Autodesk Inventor part; units mm, degrees
(part 2 of 2)
  arc A534 (23.3689, 24.3508) -> (23.2778, 24.4378) centre (0, 0) ccw
  arc A535 (23.1753, 25.0231) -> (23.2778, 24.4378) centre (23.6226, 24.7999) ccw
  arc A536 (23.5592, 25.726) -> (23.1753, 25.0231) centre (32.8115, 20.2148) ccw
  arc A537 (23.5592, 25.726) -> (23.6135, 25.8342) centre (22.847, 26.1505) ccw
  arc A538 (23.6135, 25.8342) -> (23.96, 26.7897) centre (12.8293, 30.2854) ccw
  arc A539 (23.96, 26.7897) -> (23.931, 26.8943) centre (23.8646, 26.8196) ccw
  arc A540 (23.931, 26.8943) -> (23.4386, 27.3246) centre (0, 0) ccw
  arc A541 (23.4386, 27.3246) -> (23.331, 27.3392) centre (23.3735, 27.2487) ccw
  arc A542 (23.331, 27.3392) -> (22.4306, 26.8676) centre (28.2892, 16.7785) ccw
  arc A543 (22.4306, 26.8676) -> (22.3307, 26.7993) centre (22.847, 26.1505) ccw
  arc A544 (21.6857, 26.3244) -> (22.3307, 26.7993) centre (15.6275, 35.228) ccw
  arc A545 (21.092, 26.3475) -> (21.6857, 26.3244) centre (21.4045, 26.7378) ccw
  arc A546 (21.092, 26.3475) -> (20.9935, 26.426) centre (0, 0) ccw
  arc A547 (20.8389, 26.9998) -> (20.9935, 26.426) centre (21.3045, 26.8175) ccw
  arc A548 (21.1584, 27.7342) -> (20.8389, 26.9998) centre (30.8673, 23.0746) ccw
  arc A549 (21.1584, 27.7342) -> (21.2027, 27.8469) centre (20.4109, 28.0932) ccw
  arc A550 (21.2027, 27.8469) -> (21.4621, 28.8296) centre (10.0629, 31.3135) ccw
  arc A551 (21.4621, 28.8296) -> (21.4239, 28.9312) centre (21.3644, 28.8509) ccw
  arc A552 (21.4239, 28.9312) -> (20.8949, 29.3156) centre (0, 0) ccw
  arc A553 (20.8949, 29.3156) -> (20.7864, 29.3205) centre (20.8368, 29.2342) ccw
  arc A554 (20.7864, 29.3205) -> (19.932, 28.7701) centre (26.6713, 19.2468) ccw
  arc A555 (19.932, 28.7701) -> (19.8385, 28.6931) centre (20.4109, 28.0932) ccw
  arc A556 (19.2387, 28.1624) -> (19.8385, 28.6931) centre (12.4067, 36.487) ccw
  arc A557 (18.6453, 28.1321) -> (19.2387, 28.1624) centre (18.9215, 28.5489) ccw
  arc A558 (18.6453, 28.1321) -> (18.5402, 28.2015) centre (0, 0) ccw
  arc A559 (18.3348, 28.7591) -> (18.5402, 28.2015) centre (18.8148, 28.6193) ccw
  arc A560 (18.5871, 29.5192) -> (18.3348, 28.7591) centre (28.6747, 25.7486) ccw
  arc A561 (18.5871, 29.5192) -> (18.6211, 29.6353) centre (17.8105, 29.8098) ccw
  arc A562 (18.6211, 29.6353) -> (18.7914, 30.6374) centre (7.2155, 32.0894) ccw
  arc A563 (18.7914, 30.6374) -> (18.7443, 30.7352) centre (18.6922, 30.6498) ccw
  arc A564 (18.7443, 30.7352) -> (18.1829, 31.0706) centre (0, 0) ccw
  arc A565 (18.1829, 31.0706) -> (18.0745, 31.0657) centre (18.1324, 30.9843) ccw
  arc A566 (18.0745, 31.0657) -> (17.2728, 30.4409) centre (24.8386, 21.5601) ccw
  arc A567 (17.2728, 30.4409) -> (17.1866, 30.3559) centre (17.8105, 29.8098) ccw
  arc A568 (16.6368, 29.7735) -> (17.1866, 30.3559) centre (9.0861, 37.4523) ccw
  arc A569 (16.0485, 29.6902) -> (16.6368, 29.7735) centre (16.2863, 30.1301) ccw
  arc A570 (16.0485, 29.6902) -> (15.9376, 29.7499) centre (0, 0) ccw
  arc A571 (15.683, 30.2868) -> (15.9376, 29.7499) centre (16.1737, 30.1906) ccw
  arc A572 (15.8662, 31.0665) -> (15.683, 30.2868) centre (26.2511, 28.2154) ccw
  arc A573 (15.8662, 31.0665) -> (15.8897, 31.1852) centre (15.0667, 31.2863) ccw
  arc A574 (15.8897, 31.1852) -> (15.9695, 32.1985) centre (4.31, 32.607) ccw
  arc A575 (15.9695, 32.1985) -> (15.9137, 32.2917) centre (15.8695, 32.202) ccw
  arc A576 (15.9137, 32.2917) -> (15.3246, 32.5754) centre (0, 0) ccw
  arc A577 (15.3246, 32.5754) -> (15.217, 32.5609) centre (15.282, 32.4849) ccw
  arc A578 (15.217, 32.5609) -> (14.4745, 31.8667) centre (22.806, 23.6998) ccw
  arc A579 (14.4745, 31.8667) -> (14.3964, 31.7743) centre (15.0667, 31.2863) ccw
  arc A580 (13.901, 31.145) -> (14.3964, 31.7743) centre (5.6923, 38.116) ccw
  arc A581 (13.3225, 31.0092) -> (13.901, 31.145) centre (13.5199, 31.4686) ccw
  arc A582 (13.3225, 31.0092) -> (13.2066, 31.0588) centre (0, 0) ccw
  arc A583 (12.905, 31.5707) -> (13.2066, 31.0588) centre (13.4023, 31.5189) ccw
  arc A584 (13.0175, 32.3637) -> (12.905, 31.5707) centre (23.6163, 30.4549) ccw
  arc A585 (13.0175, 32.3637) -> (13.0303, 32.484) centre (12.2015, 32.5109) ccw
  arc A586 (13.0303, 32.484) -> (13.0189, 33.5004) centre (1.3697, 32.8621) ccw
  arc A587 (13.0189, 33.5004) -> (12.9551, 33.5882) centre (12.9191, 33.4949) ccw
  arc A588 (12.9551, 33.5882) -> (12.3429, 33.8179) centre (0, 0) ccw
  arc A589 (12.3429, 33.8179) -> (12.237, 33.7938) centre (12.3086, 33.724) ccw
  arc A590 (12.237, 33.7938) -> (11.5598, 33.0359) centre (20.5897, 25.6487) ccw
  arc A591 (11.5598, 33.0359) -> (11.4902, 32.9369) centre (12.2015, 32.5109) ccw
  arc A592 (11.0532, 32.2657) -> (11.4902, 32.9369) centre (2.2527, 38.4728) ccw
  arc A593 (10.4892, 32.0786) -> (11.0532, 32.2657) centre (10.6446, 32.5539) ccw
  arc A594 (10.4892, 32.0786) -> (10.3694, 32.1176) centre (0, 0) ccw
  arc A595 (10.0231, 32.6004) -> (10.3694, 32.1176) centre (10.523, 32.5934) ccw
  arc A596 (10.0641, 33.4003) -> (10.0231, 32.6004) centre (20.7912, 32.4493) ccw
  arc A597 (10.0641, 33.4003) -> (10.066, 33.5213) centre (9.2382, 33.4738) ccw
  arc A598 (10.066, 33.5213) -> (9.9636, 34.5325) centre (-1.5815, 32.8526) ccw
  arc A599 (9.9636, 34.5325) -> (9.8921, 34.6143) centre (9.8646, 34.5181) ccw
  arc A600 (9.8921, 34.6143) -> (9.2618, 34.7882) centre (0, 0) ccw
  arc A601 (9.2618, 34.7882) -> (9.1585, 34.7547) centre (9.236, 34.6916) ccw
  arc A602 (9.1585, 34.7547) -> (8.5519, 33.9391) centre (18.2077, 27.3911) ccw
  arc A603 (8.5519, 33.9391) -> (8.4915, 33.8343) centre (9.2382, 33.4738) ccw
  arc A604 (8.1164, 33.1266) -> (8.4915, 33.8343) centre (-1.205, 38.5198) ccw
  arc A605 (7.5715, 32.8897) -> (8.1164, 33.1266) centre (7.6837, 33.377) ccw
  arc A606 (7.5715, 32.8897) -> (7.4487, 32.9178) centre (0, 0) ccw
  arc A607 (7.0604, 33.3676) -> (7.4487, 32.9178) centre (7.559, 33.4054) ccw
  arc A608 (7.0296, 34.1679) -> (7.0604, 33.3676) centre (17.7988, 34.1823) ccw
  arc A609 (7.0296, 34.1679) -> (7.0206, 34.2886) centre (6.2004, 34.1671) ccw
  arc A610 (7.0206, 34.2886) -> (6.828, 35.2866) centre (-4.52, 32.5786) ccw
  arc A611 (6.828, 35.2866) -> (6.7495, 35.3616) centre (6.7307, 35.2634) ccw
  arc A612 (6.7495, 35.3616) -> (6.1061, 35.4784) centre (0, 0) ccw
  arc A613 (6.1061, 35.4784) -> (6.0062, 35.4357) centre (6.0891, 35.3798) ccw
  arc A614 (6.0062, 35.4357) -> (5.4752, 34.5691) centre (15.6791, 28.913) ccw
  arc A615 (5.4752, 34.5691) -> (5.4244, 34.4592) centre (6.2004, 34.1671) ccw
  arc A616 (5.1143, 33.7208) -> (5.4244, 34.4592) centre (-4.6531, 38.2567) ccw
  arc A617 (4.5928, 33.436) -> (5.1143, 33.7208) centre (4.6608, 33.9314) ccw
  arc A618 (4.5928, 33.436) -> (4.4679, 33.453) centre (0, 0) ccw
  arc A619 (4.041, 33.8662) -> (4.4679, 33.453) centre (4.5341, 33.9486) ccw
  arc A620 (3.9385, 34.6605) -> (4.041, 33.8662) centre (14.6631, 35.6402) ccw
  arc A621 (3.9385, 34.6605) -> (3.9188, 34.7799) centre (3.1127, 34.5854) ccw
  arc A622 (3.9188, 34.7799) -> (3.6374, 35.7566) centre (-7.4222, 32.0423) ccw
  arc A623 (3.6374, 35.7566) -> (3.5525, 35.8243) centre (3.5426, 35.7248) ccw
  arc A624 (3.5525, 35.8243) -> (2.9013, 35.8829) centre (0, 0) ccw
  arc A625 (2.9013, 35.8829) -> (2.8056, 35.8315) centre (2.8932, 35.7832) ccw
  arc A626 (2.8056, 35.8315) -> (2.3544, 34.9207) centre (13.0242, 30.202) ccw
  arc A627 (2.3544, 34.9207) -> (2.3137, 34.8068) centre (3.1127, 34.5854) ccw
  arc A628 (2.071, 34.0435) -> (2.3137, 34.8068) centre (-8.0636, 37.6856) ccw
  arc A629 (1.5771, 33.7131) -> (2.071, 34.0435) centre (1.6005, 34.2126) ccw
  arc A630 (1.5771, 33.7131) -> (1.4513, 33.7188) centre (0, 0) ccw
  arc A631 (0.989, 34.0921) -> (1.4513, 33.7188) centre (1.4728, 34.2183) ccw
  arc A632 (0.8157, 34.874) -> (0.989, 34.0921) centre (11.4093, 36.8111) ccw
  arc A633 (0.8157, 34.874) -> (0.7853, 34.9912) centre (0, 34.7251) ccw
  arc A634 (0.7853, 34.9912) -> (0.4176, 35.9387) centre (-10.2645, 31.2479) ccw
  arc A635 (0.4176, 35.9387) -> (0.3269, 35.9985) centre (0.326, 35.8985) ccw
  arc A636 (0.3269, 35.9985) -> (-0.3269, 35.9985) centre (0, 0) ccw
  arc A637 (-0.3269, 35.9985) -> (-0.4176, 35.9387) centre (-0.326, 35.8985) ccw
  arc A638 (-0.4176, 35.9387) -> (-0.7853, 34.9912) centre (10.2645, 31.2479) ccw
  arc A639 (-0.7853, 34.9912) -> (-0.8157, 34.874) centre (0, 34.7251) ccw
  arc A640 (-0.989, 34.0921) -> (-0.8157, 34.874) centre (-11.4093, 36.8111) ccw
  arc A641 (-1.4513, 33.7188) -> (-0.989, 34.0921) centre (-1.4728, 34.2183) ccw
  arc A642 (-1.4513, 33.7188) -> (-1.5771, 33.7131) centre (0, 0) ccw
  arc A643 (-2.071, 34.0435) -> (-1.5771, 33.7131) centre (-1.6005, 34.2126) ccw
  arc A644 (-2.3137, 34.8068) -> (-2.071, 34.0435) centre (8.0636, 37.6856) ccw
  arc A645 (-2.3137, 34.8068) -> (-2.3544, 34.9207) centre (-3.1127, 34.5854) ccw
  arc A646 (-2.3544, 34.9207) -> (-2.8056, 35.8315) centre (-13.0242, 30.202) ccw
  arc A647 (-2.8056, 35.8315) -> (-2.9013, 35.8829) centre (-2.8932, 35.7832) ccw
  arc A648 (-2.9013, 35.8829) -> (-3.5525, 35.8243) centre (0, 0) ccw
  arc A649 (-3.5525, 35.8243) -> (-3.6374, 35.7566) centre (-3.5426, 35.7248) ccw
  arc A650 (-3.6374, 35.7566) -> (-3.9188, 34.7799) centre (7.4222, 32.0423) ccw
  arc A651 (-3.9188, 34.7799) -> (-3.9385, 34.6605) centre (-3.1127, 34.5854) ccw
  arc A652 (-4.041, 33.8662) -> (-3.9385, 34.6605) centre (-14.6631, 35.6402) ccw
  arc A653 (-4.4679, 33.453) -> (-4.041, 33.8662) centre (-4.5341, 33.9486) ccw
  arc A654 (-4.4679, 33.453) -> (-4.5928, 33.436) centre (0, 0) ccw
  arc A655 (-5.1143, 33.7208) -> (-4.5928, 33.436) centre (-4.6608, 33.9314) ccw
  arc A656 (-5.4244, 34.4592) -> (-5.1143, 33.7208) centre (4.6531, 38.2567) ccw
  arc A657 (-5.4244, 34.4592) -> (-5.4752, 34.5691) centre (-6.2004, 34.1671) ccw
  arc A658 (-5.4752, 34.5691) -> (-6.0062, 35.4357) centre (-15.6791, 28.913) ccw
  arc A659 (-6.0062, 35.4357) -> (-6.1061, 35.4784) centre (-6.0891, 35.3798) ccw
  arc A660 (-6.1061, 35.4784) -> (-6.7495, 35.3616) centre (0, 0) ccw
  arc A661 (-6.7495, 35.3616) -> (-6.828, 35.2866) centre (-6.7307, 35.2634) ccw
  arc A662 (-6.828, 35.2866) -> (-7.0206, 34.2886) centre (4.52, 32.5786) ccw
  arc A663 (-7.0206, 34.2886) -> (-7.0296, 34.1679) centre (-6.2004, 34.1671) ccw
  arc A664 (-7.0604, 33.3676) -> (-7.0296, 34.1679) centre (-17.7988, 34.1823) ccw
  arc A665 (-7.4487, 32.9178) -> (-7.0604, 33.3676) centre (-7.559, 33.4054) ccw
  arc A666 (-7.4487, 32.9178) -> (-7.5715, 32.8897) centre (0, 0) ccw
  arc A667 (-8.1164, 33.1266) -> (-7.5715, 32.8897) centre (-7.6837, 33.377) ccw
  arc A668 (-8.4915, 33.8343) -> (-8.1164, 33.1266) centre (1.205, 38.5198) ccw
  arc A669 (-8.4915, 33.8343) -> (-8.5519, 33.9391) centre (-9.2382, 33.4738) ccw
  arc A670 (-8.5519, 33.9391) -> (-9.1585, 34.7547) centre (-18.2077, 27.3911) ccw
  arc A671 (-9.1585, 34.7547) -> (-9.2618, 34.7882) centre (-9.236, 34.6916) ccw
  arc A672 (-9.2618, 34.7882) -> (-9.8921, 34.6143) centre (0, 0) ccw
  arc A673 (-9.8921, 34.6143) -> (-9.9636, 34.5325) centre (-9.8646, 34.5181) ccw
  arc A674 (-9.9636, 34.5325) -> (-10.066, 33.5213) centre (1.5815, 32.8526) ccw
  arc A675 (-10.066, 33.5213) -> (-10.0641, 33.4003) centre (-9.2382, 33.4738) ccw
  arc A676 (-10.0231, 32.6004) -> (-10.0641, 33.4003) centre (-20.7912, 32.4493) ccw
  arc A677 (-10.3694, 32.1176) -> (-10.0231, 32.6004) centre (-10.523, 32.5934) ccw
  arc A678 (-10.3694, 32.1176) -> (-10.4892, 32.0786) centre (0, 0) ccw
  arc A679 (-11.0532, 32.2657) -> (-10.4892, 32.0786) centre (-10.6446, 32.5539) ccw
  arc A680 (-11.4902, 32.9369) -> (-11.0532, 32.2657) centre (-2.2527, 38.4728) ccw
  arc A681 (-11.4902, 32.9369) -> (-11.5598, 33.0359) centre (-12.2015, 32.5109) ccw
  arc A682 (-11.5598, 33.0359) -> (-12.237, 33.7938) centre (-20.5897, 25.6487) ccw
  arc A683 (-12.237, 33.7938) -> (-12.3429, 33.8179) centre (-12.3086, 33.724) ccw
  arc A684 (-12.3429, 33.8179) -> (-12.9551, 33.5882) centre (0, 0) ccw
  arc A685 (-12.9551, 33.5882) -> (-13.0189, 33.5004) centre (-12.9191, 33.4949) ccw
  arc A686 (-13.0189, 33.5004) -> (-13.0303, 32.484) centre (-1.3697, 32.8621) ccw
  arc A687 (-13.0303, 32.484) -> (-13.0175, 32.3637) centre (-12.2015, 32.5109) ccw
  arc A688 (-12.905, 31.5707) -> (-13.0175, 32.3637) centre (-23.6163, 30.4549) ccw
  arc A689 (-13.2066, 31.0588) -> (-12.905, 31.5707) centre (-13.4023, 31.5189) ccw
  arc A690 (-13.2066, 31.0588) -> (-13.3225, 31.0092) centre (0, 0) ccw
  arc A691 (-13.901, 31.145) -> (-13.3225, 31.0092) centre (-13.5199, 31.4686) ccw
  arc A692 (-14.3964, 31.7743) -> (-13.901, 31.145) centre (-5.6923, 38.116) ccw
  arc A693 (-14.3964, 31.7743) -> (-14.4745, 31.8667) centre (-15.0667, 31.2863) ccw
  arc A694 (-14.4745, 31.8667) -> (-15.217, 32.5609) centre (-22.806, 23.6998) ccw
  arc A695 (-15.217, 32.5609) -> (-15.3246, 32.5754) centre (-15.282, 32.4849) ccw
  arc A696 (-15.3246, 32.5754) -> (-15.9137, 32.2917) centre (0, 0) ccw
  arc A697 (-15.9137, 32.2917) -> (-15.9695, 32.1985) centre (-15.8695, 32.202) ccw
  arc A698 (-15.9695, 32.1985) -> (-15.8897, 31.1852) centre (-4.31, 32.607) ccw
  arc A699 (-15.8897, 31.1852) -> (-15.8662, 31.0665) centre (-15.0667, 31.2863) ccw
  arc A700 (-15.683, 30.2868) -> (-15.8662, 31.0665) centre (-26.2511, 28.2154) ccw
  arc A701 (-15.9376, 29.7499) -> (-15.683, 30.2868) centre (-16.1737, 30.1906) ccw
  arc A702 (-15.9376, 29.7499) -> (-16.0485, 29.6902) centre (0, 0) ccw
  arc A703 (-16.6368, 29.7735) -> (-16.0485, 29.6902) centre (-16.2863, 30.1301) ccw
  arc A704 (-17.1866, 30.3559) -> (-16.6368, 29.7735) centre (-9.0861, 37.4523) ccw
  arc A705 (-17.1866, 30.3559) -> (-17.2728, 30.4409) centre (-17.8105, 29.8098) ccw
  arc A706 (-17.2728, 30.4409) -> (-18.0745, 31.0657) centre (-24.8386, 21.5601) ccw
  arc A707 (-18.0745, 31.0657) -> (-18.1829, 31.0706) centre (-18.1324, 30.9843) ccw
  arc A708 (-18.1829, 31.0706) -> (-18.7443, 30.7352) centre (0, 0) ccw
  arc A709 (-18.7443, 30.7352) -> (-18.7914, 30.6374) centre (-18.6922, 30.6498) ccw
  arc A710 (-18.7914, 30.6374) -> (-18.6211, 29.6353) centre (-7.2155, 32.0894) ccw
  arc A711 (-18.6211, 29.6353) -> (-18.5871, 29.5192) centre (-17.8105, 29.8098) ccw
  arc A712 (-18.3348, 28.7591) -> (-18.5871, 29.5192) centre (-28.6747, 25.7486) ccw
  arc A713 (-18.5402, 28.2015) -> (-18.3348, 28.7591) centre (-18.8148, 28.6193) ccw
  arc A714 (-18.5402, 28.2015) -> (-18.6453, 28.1321) centre (0, 0) ccw
  arc A715 (-19.2387, 28.1624) -> (-18.6453, 28.1321) centre (-18.9215, 28.5489) ccw
  arc A716 (-19.8385, 28.6931) -> (-19.2387, 28.1624) centre (-12.4067, 36.487) ccw
  arc A717 (-19.8385, 28.6931) -> (-19.932, 28.7701) centre (-20.4109, 28.0932) ccw
  arc A718 (-19.932, 28.7701) -> (-20.7864, 29.3205) centre (-26.6713, 19.2468) ccw
  arc A719 (-20.7864, 29.3205) -> (-20.8949, 29.3156) centre (-20.8368, 29.2342) ccw
  arc A720 (-20.8949, 29.3156) -> (-21.4239, 28.9312) centre (0, 0) ccw
  arc A721 (-21.4239, 28.9312) -> (-21.4621, 28.8296) centre (-21.3644, 28.8509) ccw
  arc A722 (-21.4621, 28.8296) -> (-21.2027, 27.8469) centre (-10.0629, 31.3135) ccw
  arc A723 (-21.2027, 27.8469) -> (-21.1584, 27.7342) centre (-20.4109, 28.0932) ccw
  arc A724 (-20.8389, 26.9998) -> (-21.1584, 27.7342) centre (-30.8673, 23.0746) ccw
  arc A725 (-20.9935, 26.426) -> (-20.8389, 26.9998) centre (-21.3045, 26.8175) ccw
  arc A726 (-20.9935, 26.426) -> (-21.092, 26.3475) centre (0, 0) ccw
  arc A727 (-21.6857, 26.3244) -> (-21.092, 26.3475) centre (-21.4045, 26.7378) ccw
  arc A728 (-22.3307, 26.7993) -> (-21.6857, 26.3244) centre (-15.6275, 35.228) ccw
  arc A729 (-22.3307, 26.7993) -> (-22.4306, 26.8676) centre (-22.847, 26.1505) ccw
  arc A730 (-22.4306, 26.8676) -> (-23.331, 27.3392) centre (-28.2892, 16.7785) ccw
  arc A731 (-23.331, 27.3392) -> (-23.4386, 27.3246) centre (-23.3735, 27.2487) ccw
  arc A732 (-23.4386, 27.3246) -> (-23.931, 26.8943) centre (0, 0) ccw
  arc A733 (-23.931, 26.8943) -> (-23.96, 26.7897) centre (-23.8646, 26.8196) ccw
  arc A734 (-23.96, 26.7897) -> (-23.6135, 25.8342) centre (-12.8293, 30.2854) ccw
  arc A735 (-23.6135, 25.8342) -> (-23.5592, 25.726) centre (-22.847, 26.1505) ccw
  arc A736 (-23.1753, 25.0231) -> (-23.5592, 25.726) centre (-32.8115, 20.2148) ccw
  arc A737 (-23.2778, 24.4378) -> (-23.1753, 25.0231) centre (-23.6226, 24.7999) ccw
  arc A738 (-23.2778, 24.4378) -> (-23.3689, 24.3508) centre (0, 0) ccw
  arc A739 (-23.9582, 24.2746) -> (-23.3689, 24.3508) centre (-23.7151, 24.7115) ccw
  arc A740 (-24.6431, 24.6897) -> (-23.9582, 24.2746) centre (-18.7224, 33.6854) ccw
  arc A741 (-24.6431, 24.6897) -> (-24.7487, 24.7487) centre (-25.0992, 23.9973) ccw
  arc A742 (-24.7487, 24.7487) -> (-25.6877, 25.1378) centre (-29.6793, 14.1751) ccw
  arc A743 (-25.6877, 25.1378) -> (-25.7936, 25.1135) centre (-25.722, 25.0438) ccw
  arc A744 (-25.7936, 25.1135) -> (-26.2455, 24.6409) centre (0, 0) ccw
  arc A745 (-26.2455, 24.6409) -> (-26.2649, 24.5341) centre (-26.1726, 24.5725) ccw
  arc A746 (-26.2649, 24.5341) -> (-25.8342, 23.6135) centre (-15.4924, 29.0134) ccw
  arc A747 (-25.8342, 23.6135) -> (-25.7705, 23.5106) centre (-25.0992, 23.9973) ccw
  arc A748 (-25.325, 22.845) -> (-25.7705, 23.5106) centre (-34.4914, 17.1922) ccw
  arc A749 (-25.3747, 22.2528) -> (-25.325, 22.845) centre (-25.7506, 22.5825) ccw
  arc A750 (-25.3747, 22.2528) -> (-25.4576, 22.158) centre (0, 0) ccw
  arc A751 (-26.0377, 22.0293) -> (-25.4576, 22.158) centre (-25.8347, 22.4862) ccw
  arc A752 (-26.757, 22.3813) -> (-26.0377, 22.0293) centre (-21.6665, 31.8715) ccw
  arc A753 (-26.757, 22.3813) -> (-26.8676, 22.4306) centre (-27.1492, 21.6508) ccw
  arc A754 (-26.8676, 22.4306) -> (-27.8377, 22.7339) centre (-30.8305, 11.4577) ccw
  arc A755 (-27.8377, 22.7339) -> (-27.9409, 22.7003) centre (-27.8633, 22.6373) ccw
  arc A756 (-27.9409, 22.7003) -> (-28.3486, 22.1891) centre (0, 0) ccw
  arc A757 (-28.3486, 22.1891) -> (-28.3584, 22.0809) centre (-28.2699, 22.1275) ccw
  arc A758 (-28.3584, 22.0809) -> (-27.8469, 21.2027) centre (-18.0308, 27.5079) ccw
  arc A759 (-27.8469, 21.2027) -> (-27.7742, 21.1059) centre (-27.1492, 21.6508) ccw
  arc A760 (-27.2709, 20.4829) -> (-27.7742, 21.1059) centre (-35.8937, 14.0312) ccw
  arc A761 (-27.2672, 19.8887) -> (-27.2709, 20.4829) centre (-27.6712, 20.1833) ccw
  arc A762 (-27.2672, 19.8887) -> (-27.3413, 19.7868) centre (0, 0) ccw
  arc A763 (-27.9075, 19.6066) -> (-27.3413, 19.7868) centre (-27.7464, 20.0799) ccw
  arc A764 (-28.6556, 19.8928) -> (-27.9075, 19.6066) centre (-24.4362, 29.801) ccw
  arc A765 (-28.6556, 19.8928) -> (-28.7701, 19.932) centre (-28.9807, 19.13) ccw
  arc A766 (-28.7701, 19.932) -> (-29.7634, 20.1471) centre (-31.7334, 8.6479) ccw
  arc A767 (-29.7634, 20.1471) -> (-29.8633, 20.1043) centre (-29.7803, 20.0485) ccw
  arc A768 (-29.8633, 20.1043) -> (-30.2235, 19.5586) centre (0, 0) ccw
  arc A769 (-30.2235, 19.5586) -> (-30.2236, 19.45) centre (-30.1396, 19.5043) ccw
  arc A770 (-30.2236, 19.45) -> (-29.6353, 18.6211) centre (-20.424, 25.7809) ccw
  arc A771 (-29.6353, 18.6211) -> (-29.5543, 18.5312) centre (-28.9807, 19.13) ccw
  arc A772 (-28.9971, 17.9559) -> (-29.5543, 18.5312) centre (-37.0069, 10.7572) ccw
  arc A773 (-28.9403, 17.3644) -> (-28.9971, 17.9559) centre (-29.369, 17.6216) ccw
  arc A774 (-28.9403, 17.3644) -> (-29.0049, 17.2562) centre (0, 0) ccw
  arc A775 (-29.5527, 17.026) -> (-29.0049, 17.2562) centre (-29.4346, 17.5119) ccw
  arc A776 (-30.3234, 17.244) -> (-29.5527, 17.026) centre (-27.0092, 27.4906) ccw
  arc A777 (-30.3234, 17.244) -> (-30.4409, 17.2728) centre (-30.5788, 16.4552) ccw
  arc A778 (-30.4409, 17.2728) -> (-31.4496, 17.398) centre (-32.3808, 5.7685) ccw
  arc A779 (-31.4496, 17.398) -> (-31.5452, 17.3465) centre (-31.4576, 17.2983) ccw
  arc A780 (-31.5452, 17.3465) -> (-31.8551, 16.7707) centre (0, 0) ccw
  arc A781 (-31.8551, 16.7707) -> (-31.8454, 16.6625) centre (-31.7666, 16.7241) ccw
  arc A782 (-31.8454, 16.6625) -> (-31.1852, 15.8897) centre (-22.6528, 23.8463) ccw
  arc A783 (-31.1852, 15.8897) -> (-31.0964, 15.8074) centre (-30.5788, 16.4552) ccw
  arc A784 (-30.49, 15.2843) -> (-31.0964, 15.8074) centre (-37.8222, 7.3967) ccw
  arc A785 (-30.3803, 14.7003) -> (-30.49, 15.2843) centre (-30.8304, 14.9181) ccw
  arc A786 (-30.3803, 14.7003) -> (-30.435, 14.5868) centre (0, 0) ccw
  arc A787 (-30.9599, 14.3084) -> (-30.435, 14.5868) centre (-30.8859, 14.8029) ccw
  arc A788 (-31.747, 14.4564) -> (-30.9599, 14.3084) centre (-29.3647, 24.9588) ccw
  arc A789 (-31.747, 14.4564) -> (-31.8667, 14.4745) centre (-31.9307, 13.6479) ccw
  arc A790 (-31.8667, 14.4745) -> (-32.8825, 14.5088) centre (-32.7676, 2.8427) ccw
  arc A791 (-32.8825, 14.5088) -> (-32.9731, 14.449) centre (-32.8815, 14.4088) ccw
  arc A792 (-32.9731, 14.449) -> (-33.2301, 13.8477) centre (0, 0) ccw
  arc A793 (-33.2301, 13.8477) -> (-33.2108, 13.7408) centre (-33.1378, 13.8092) ccw
  arc A794 (-33.2108, 13.7408) -> (-32.484, 13.0303) centre (-24.6991, 21.7197) ccw
  arc A795 (-32.484, 13.0303) -> (-32.3882, 12.9563) centre (-31.9307, 13.6479) ccw
  arc A796 (-31.7373, 12.4897) -> (-32.3882, 12.9563) centre (-38.333, 3.9765) ccw
  arc A797 (-31.5757, 11.9179) -> (-31.7373, 12.4897) centre (-32.0435, 12.0944) ccw
  arc A798 (-31.5757, 11.9179) -> (-31.62, 11.7999) centre (0, 0) ccw
  arc A799 (-32.1179, 11.4756) -> (-31.62, 11.7999) centre (-32.0885, 11.9747) ccw
  arc A800 (-32.9151, 11.5524) -> (-32.1179, 11.4756) centre (-31.4838, 22.2261) ccw
  arc A801 (-32.9151, 11.5524) -> (-33.0359, 11.5598) centre (-33.0256, 10.7307) ccw
  arc A802 (-33.0359, 11.5598) -> (-34.0507, 11.5028) centre (-32.8905, -0.106) ccw
  arc A803 (-34.0507, 11.5028) -> (-34.1356, 11.4351) centre (-34.0408, 11.4033) ccw
  arc A804 (-34.1356, 11.4351) -> (-34.3377, 10.8132) centre (0, 0) ccw
  arc A805 (-34.3377, 10.8132) -> (-34.3088, 10.7085) centre (-34.2423, 10.7832) ccw
  arc A806 (-34.3088, 10.7085) -> (-33.5213, 10.066) centre (-26.5467, 19.4183) ccw
  arc A807 (-33.5213, 10.066) -> (-33.4192, 10.0009) centre (-33.0256, 10.7307) ccw
  arc A808 (-32.7291, 9.5945) -> (-33.4192, 10.0009) centre (-38.5351, 0.5244) ccw
  arc A809 (-32.5169, 9.0395) -> (-32.7291, 9.5945) centre (-32.9987, 9.1734) ccw
  arc A810 (-32.5169, 9.0395) -> (-32.5504, 8.918) centre (0, 0) ccw
  arc A811 (-33.0173, 8.5504) -> (-32.5504, 8.918) centre (-33.0327, 9.0501) ccw
  arc A812 (-33.8182, 8.5554) -> (-33.0173, 8.5504) centre (-33.3494, 19.3145) ccw
  arc A813 (-33.8182, 8.5554) -> (-33.9391, 8.5519) centre (-33.8545, 7.7271) ccw
  arc A814 (-33.9391, 8.5519) -> (-34.9447, 8.4042) centre (-32.7486, -3.0538) ccw
  arc A815 (-34.9447, 8.4042) -> (-35.0232, 8.3292) centre (-34.9259, 8.306) ccw
  arc A816 (-35.0232, 8.3292) -> (-35.1687, 7.6917) centre (0, 0) ccw
  arc A817 (-35.1687, 7.6917) -> (-35.1306, 7.59) centre (-35.071, 7.6703) ccw
  arc A818 (-35.1306, 7.59) -> (-34.2886, 7.0206) centre (-28.1804, 16.9605) ccw
  arc A819 (-34.2886, 7.0206) -> (-34.1812, 6.965) centre (-33.8545, 7.7271) ccw
  arc A820 (-33.4574, 6.622) -> (-34.1812, 6.965) centre (-38.427, -2.932) ccw
  arc A821 (-33.1963, 6.0883) -> (-33.4574, 6.622) centre (-33.6881, 6.1785) ccw
  arc A822 (-33.1963, 6.0883) -> (-33.2188, 5.9643) centre (0, 0) ccw
  arc A823 (-33.6508, 5.5563) -> (-33.2188, 5.9643) centre (-33.7109, 6.0527) ccw
  arc A824 (-34.4489, 5.4896) -> (-33.6508, 5.5563) centre (-34.9465, 16.2473) ccw
  arc A825 (-34.4489, 5.4896) -> (-34.5691, 5.4752) centre (-34.4109, 4.6613) ccw
  arc A826 (-34.5691, 5.4752) -> (-35.5574, 5.238) centre (-32.343, -5.9771) ccw
  arc A827 (-35.5574, 5.238) -> (-35.6288, 5.1562) centre (-35.5299, 5.1419) ccw
  arc A828 (-35.6288, 5.1562) -> (-35.7166, 4.5082) centre (0, 0) ccw
  arc A829 (-35.7166, 4.5082) -> (-35.6695, 4.4104) centre (-35.6174, 4.4957) ccw
  arc A830 (-35.6695, 4.4104) -> (-34.7799, 3.9188) centre (-29.5873, 14.3661) ccw
  arc A831 (-34.7799, 3.9188) -> (-34.6679, 3.8729) centre (-34.4109, 4.6613) ccw
  arc A832 (-33.9163, 3.5963) -> (-34.6679, 3.8729) centre (-38.0095, -6.3647) ccw
  arc A833 (-33.6084, 3.0881) -> (-33.9163, 3.5963) centre (-34.1063, 3.1338) ccw
  arc A834 (-33.6084, 3.0881) -> (-33.6197, 2.9626) centre (0, 0) ccw
  arc A835 (-34.0134, 2.5175) -> (-33.6197, 2.9626) centre (-34.1178, 3.0065) ccw
  arc A836 (-34.8023, 2.3795) -> (-34.0134, 2.5175) centre (-36.2622, 13.0493) ccw
  arc A837 (-34.8023, 2.3795) -> (-34.9207, 2.3544) centre (-34.6902, 1.5579) ccw
  arc A838 (-34.9207, 2.3544) -> (-35.8838, 2.0296) centre (-31.677, -8.8523) ccw
  arc A839 (-35.8838, 2.0296) -> (-35.9476, 1.9417) centre (-35.8477, 1.9363) ccw
  arc A840 (-35.9476, 1.9417) -> (-35.9769, 1.2884) centre (0, 0) ccw
  constraints: 1680 point on circle, 841 centre point
extrude "Extrusion1" cut sketch "_____12" against normal blind 10
sketch "Sketch3" plane through (0, 0, -20) normal (0, 0, -1) x (-1, 0, 0)
  point P0 (0, 0)
hole "Hole1" at (0, 0, -20) direction (0, 0, 1) diameter 10 depth 20
sketch "_____5" plane through (0, 0, 0) normal (1, 0, 0) x (0, 0, -1)
  line L0 (500, 0) -> (-500, 0)
  line L1 (19.7, 5) -> (20, 5)
  line L2 (20, 5) -> (20, 5.3)
  line L3 (20, 5.3) -> (19.7, 5)
  constraints: 8 end point
revolve "Revolution2" cut sketch "_____5" angle 360 about axis through (0, 0, -500) along (0, 0, -1)
sketch "_____13" plane through (0, 0, 0) normal (1, 0, 0) x (0, 0, -1)
  line L0 (500, 0) -> (-500, 0)
  line L1 (0, 5.3) -> (0, 5)
  line L2 (0, 5) -> (0.3, 5)
  line L3 (0.3, 5) -> (0, 5.3)
  constraints: 8 end point
revolve "Revolution3" cut sketch "_____13" angle 360 about axis through (0, 0, -500) along (0, 0, -1)
sketch "Sketch_4" plane through (0, 0, -16) normal (0, 0, 1) x (1, 0, 0)
  line L0 (0, 20) -> (0, 0)
  line L1 (0, 0) -> (-1.621, 0)
  line L2 (-1.621, 0) -> (-1.621, 19.621)
  line L3 (-1.621, 19.621) -> (-2, 20)
  line L4 (-2, 20) -> (0, 20)
  line L5 (0, 20) -> (0, 0)
  constraints: 12 end point
revolve "Revolution4" cut sketch "Sketch_4" angle 360 about axis through (0, 20, -16) along (0, 1, 0)
thread "Thread1" size "M4x0.7" class "6H" standard "ISO Metric profile" full length
sketch "Sketch7" plane through (0, 0, -20) normal (0, 0, -1) x (-1, 0, 0)
  point P0 (-10.6066, 10.6066)
hole "Hole2" at (10.6066, 10.6066, -20) direction (0, 0, 1) diameter 3 depth 20
pattern_linear "Rectangular Pattern1" count 2 spacing 21.2132 along (-1, 0, 0) count 2 spacing 21.2132 along (0, -1, 0) of "Hole2"
ref_plane "gear_to_screw_XY" through (0, 5, -16) normal (0, 1, 0) x (1, 0, 0)
ref_plane "gear_to_screw_YZ" through (0, 5, -16) normal (1, 0, 0) x (0, 0, -1)
ref_plane "gear_to_screw_ZX" through (0, 5, -16) normal (0, 0, -1) x (0, 1, 0)
body "Solid1"
